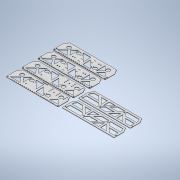
# Autodesk Inventor part: Jsun Chassi Cutout Only Outside
Saved by Autodesk Inventor 2021 (Build 250183000, 183)
## iProperties
Created: 2020-10-31
Part Number: Jsun Chassi Cutout Only Outside
Material: Generic
Document SubType Name: Modeling
Designer: deli
Density: 1 g/cm^3
Appearance: Default
Author: deli
Autodesk Inventor part; units mm, degrees
ref_plane "YZ Plane" through (0, 0, 0) normal (1, 0, 0) x (0, 1, 0)
ref_plane "XZ Plane" through (0, 0, 0) normal (0, 1, 0) x (-1, 0, 0)
ref_plane "XY Plane" through (0, 0, 0) normal (0, 0, 1) x (1, 0, 0)
sketch "Sketch1" plane through (0, 0, 0) normal (0, 1, 0) x (-1, 0, 0)
  line L0 (21, 21.4009) -> (-995, 21.4009)
  line L1 (-995, 21.4009) -> (-995, -486.5991)
  line L2 (-995, -486.5991) -> (21, -486.5991)
  line L3 (21, -486.5991) -> (21, 21.4009)
  point P0 (0, 0)
  dimension "d0" = 1016
  dimension "d1" = 508
  constraints: 8 end point, 2 parallel, 1 horizontal, 1 perpendicular
  measures "d0" distance of L2.end L1.end
  measures "d1" distance of L1.end L0.end
extrude "Extrusion1" add sketch "Sketch1" along normal blind 3.175
sketch "Sketch2" plane through (0, 3.175, 0) normal (0, 1, 0) x (1, 0, 0)
  line L0 (548.8088, 46.8923) -> (501.9154, 93.7857)
  line L1 (501.9154, 93.7857) -> (548.8088, 93.7857)
  line L2 (548.8088, 93.7857) -> (548.8088, 46.8923)
  line L3 (686.6568, 13.7857) -> (636.4088, 13.7857)
  line L4 (636.4088, 13.7857) -> (686.6568, 61.3603)
  line L5 (686.6568, 61.3603) -> (686.6568, 13.7857)
  line L6 (807.6588, 61.2857) -> (722.2634, 61.2857)
  line L7 (722.2634, 61.2857) -> (701.6568, 81.8923)
  line L8 (701.6568, 81.8923) -> (701.6568, 93.7857)
  line L9 (701.6568, 93.7857) -> (796.2302, 93.7857)
  line L10 (796.2302, 93.7857) -> (807.6588, 73.7857)
  line L11 (807.6588, 73.7857) -> (807.6588, 61.2857)
  line L12 (686.6568, 93.7857) -> (686.6568, 81.8923)
  line L13 (686.6568, 81.8923) -> (666.0502, 61.2857)
  line L14 (666.0502, 61.2857) -> (599.4154, 61.2857)
  line L15 (599.4154, 61.2857) -> (631.9154, 93.7857)
  line L16 (631.9154, 93.7857) -> (686.6568, 93.7857)
  line L17 (442.6815, 93.7857) -> (480.7022, 93.7857)
  line L18 (480.7022, 93.7857) -> (513.2022, 61.2857)
  line L19 (513.2022, 61.2857) -> (431.2588, 61.2857)
  line L20 (431.2588, 61.2857) -> (431.2588, 73.7857)
  line L21 (431.2588, 73.7857) -> (442.6815, 93.7857)
  line L22 (563.8088, 93.7857) -> (610.7022, 93.7857)
  line L23 (610.7022, 93.7857) -> (563.8088, 46.8923)
  line L24 (563.8088, 46.8923) -> (563.8088, 93.7857)
  line L25 (701.6568, 13.7857) -> (701.6568, 60.6791)
  line L26 (701.6568, 60.6791) -> (748.5502, 13.7857)
  line L27 (748.5502, 13.7857) -> (701.6568, 13.7857)
  line L28 (807.6588, 13.7857) -> (769.7634, 13.7857)
  line L29 (769.7634, 13.7857) -> (737.2634, 46.2857)
  line L30 (737.2634, 46.2857) -> (807.6588, 46.2857)
  line L31 (807.6588, 46.2857) -> (807.6588, 13.7857)
  line L32 (563.8088, 13.7857) -> (563.8088, 25.6791)
  line L33 (563.8088, 25.6791) -> (584.4154, 46.2857)
  line L34 (584.4154, 46.2857) -> (651.0502, 46.2857)
  line L35 (651.0502, 46.2857) -> (618.5502, 13.7857)
  line L36 (618.5502, 13.7857) -> (563.8088, 13.7857)
  line L37 (548.8088, 13.7857) -> (431.2588, 13.7857)
  line L38 (431.2588, 13.7857) -> (431.2588, 46.2857)
  line L39 (431.2588, 46.2857) -> (528.2022, 46.2857)
  line L40 (528.2022, 46.2857) -> (548.8088, 25.6791)
  line L41 (548.8088, 25.6791) -> (548.8088, 13.7857)
  circle A0 centre (556.3088, 28.7857) radius 3.5
  circle A1 centre (694.1568, 78.7857) radius 3.5
  circle A2 centre (423.1288, 20.1607) radius 3.5
  circle A3 centre (815.7882, 20.1789) radius 3.5
  line L42 (419.4482, -1.2143) -> (819.4793, -1.2143)
  line L43 (819.4793, -1.2143) -> (822.6588, 4.2927)
  line L44 (822.6588, 4.2927) -> (822.6588, 73.7857)
  line L45 (822.6588, 73.7857) -> (802.6588, 108.7857)
  line L46 (802.6588, 108.7857) -> (436.2486, 108.7857)
  line L47 (436.2486, 108.7857) -> (416.2588, 73.7857)
  line L48 (416.2588, 73.7857) -> (416.2588, 4.3099)
  line L49 (416.2588, 4.3099) -> (419.4482, -1.2143)
  line L50 (822.6588, 200.7857) -> (802.6588, 235.7857)
  line L51 (610.7022, 220.7857) -> (563.8088, 173.8923)
  line L52 (563.8088, 220.7857) -> (610.7022, 220.7857)
  line L53 (563.8088, 173.8923) -> (563.8088, 220.7857)
  line L54 (618.5502, 140.7857) -> (563.8088, 140.7857)
  line L55 (563.8088, 152.6791) -> (584.4154, 173.2857)
  line L56 (563.8088, 140.7857) -> (563.8088, 152.6791)
  circle A4 centre (556.3088, 155.7857) radius 3.5
  line L57 (548.8088, 152.6791) -> (548.8088, 140.7857)
  line L58 (528.2022, 173.2857) -> (548.8088, 152.6791)
  line L59 (548.8088, 220.7857) -> (548.8088, 173.8923)
  line L60 (548.8088, 173.8923) -> (501.9154, 220.7857)
  line L61 (501.9154, 220.7857) -> (548.8088, 220.7857)
  line L62 (480.7022, 220.7857) -> (513.2022, 188.2857)
  line L63 (442.6815, 220.7857) -> (480.7022, 220.7857)
  line L64 (548.8088, 140.7857) -> (431.2588, 140.7857)
  line L65 (431.2588, 173.2857) -> (528.2022, 173.2857)
  line L66 (513.2022, 188.2857) -> (431.2588, 188.2857)
  line L67 (431.2588, 188.2857) -> (431.2588, 200.7857)
  line L68 (431.2588, 140.7857) -> (431.2588, 173.2857)
  circle A5 centre (423.1288, 147.1607) radius 3.5
  line L69 (416.2588, 131.3099) -> (419.4482, 125.7857)
  line L70 (416.2588, 200.7857) -> (416.2588, 131.3099)
  line L71 (436.2486, 235.7857) -> (416.2588, 200.7857)
  line L72 (431.2588, 200.7857) -> (442.6815, 220.7857)
  line L73 (796.2302, 220.7857) -> (807.6588, 200.7857)
  line L74 (807.6588, 200.7857) -> (807.6588, 188.2857)
  circle A6 centre (815.7882, 147.1789) radius 3.5
  line L75 (822.6588, 131.2927) -> (822.6588, 200.7857)
  line L76 (819.4793, 125.7857) -> (822.6588, 131.2927)
  line L77 (807.6588, 173.2857) -> (807.6588, 140.7857)
  line L78 (737.2634, 173.2857) -> (807.6588, 173.2857)
  line L79 (807.6588, 140.7857) -> (769.7634, 140.7857)
  line L80 (807.6588, 188.2857) -> (722.2634, 188.2857)
  line L81 (701.6568, 220.7857) -> (796.2302, 220.7857)
  line L82 (769.7634, 140.7857) -> (737.2634, 173.2857)
  line L83 (722.2634, 188.2857) -> (701.6568, 208.8923)
  line L84 (701.6568, 187.6791) -> (748.5502, 140.7857)
  line L85 (748.5502, 140.7857) -> (701.6568, 140.7857)
  line L86 (701.6568, 140.7857) -> (701.6568, 187.6791)
  line L87 (701.6568, 208.8923) -> (701.6568, 220.7857)
  line L88 (599.4154, 188.2857) -> (631.9154, 220.7857)
  line L89 (584.4154, 173.2857) -> (651.0502, 173.2857)
  line L90 (802.6588, 235.7857) -> (436.2486, 235.7857)
  line L91 (419.4482, 125.7857) -> (819.4793, 125.7857)
  line L92 (666.0502, 188.2857) -> (599.4154, 188.2857)
  line L93 (651.0502, 173.2857) -> (618.5502, 140.7857)
  line L94 (631.9154, 220.7857) -> (686.6568, 220.7857)
  line L95 (686.6568, 140.7857) -> (636.4088, 140.7857)
  line L96 (636.4088, 140.7857) -> (686.6568, 188.3603)
  line L97 (686.6568, 188.3603) -> (686.6568, 140.7857)
  line L98 (686.6568, 208.8923) -> (666.0502, 188.2857)
  line L99 (686.6568, 220.7857) -> (686.6568, 208.8923)
  circle A7 centre (694.1568, 205.7857) radius 3.5
  circle A8 centre (367.8668, 73.0303) radius 2
  circle A9 centre (367.8668, 81.0303) radius 2
  circle A10 centre (367.8668, 65.0303) radius 2
  circle A11 centre (367.8668, 89.0303) radius 2
  circle A12 centre (367.8668, 57.0303) radius 2
  line L100 (185.8606, 84.0272) -> (190.0041, 79.8837)
  line L101 (190.0041, 79.8837) -> (190.0041, 23.4497)
  line L102 (190.0041, 23.4497) -> (129.4266, 84.0272)
  line L103 (129.4266, 84.0272) -> (185.8606, 84.0272)
  line L104 (205.0041, 64.8837) -> (265.5816, 4.3062)
  line L105 (265.5816, 4.3062) -> (209.1476, 4.3062)
  line L106 (209.1476, 4.3062) -> (205.0041, 8.4497)
  line L107 (205.0041, 8.4497) -> (205.0041, 64.8837)
  line L108 (93.7196, 15.6062) -> (59.7512, 53.8845)
  line L109 (59.7512, 53.8845) -> (93.7196, 84.0272)
  line L110 (93.7196, 84.0272) -> (93.7196, 15.6062)
  line L111 (312.2569, 4.3062) -> (346.6857, 38.2085)
  line L112 (346.6857, 38.2085) -> (380.0696, 4.3062)
  line L113 (380.0696, 4.3062) -> (312.2569, 4.3062)
  line L114 (3.8839, 4.3093) -> (48.5317, 43.9286)
  line L115 (48.5317, 43.9286) -> (83.6949, 4.3093)
  line L116 (83.6949, 4.3093) -> (3.8839, 4.3093)
  circle A13 centre (311.8668, 73.0303) radius 2
  circle A14 centre (255.8668, 65.0303) radius 2
  circle A15 centre (207.8668, 94.0303) radius 2
  circle A16 centre (175.8668, 94.0303) radius 2
  circle A17 centre (199.8668, 94.0303) radius 2
  circle A18 centre (255.8668, 73.0303) radius 2
  circle A19 centre (311.8668, 81.0303) radius 2
  circle A20 centre (311.8668, 65.0303) radius 2
  circle A21 centre (255.8668, 57.0303) radius 2
  circle A22 centre (255.8668, 81.0303) radius 2
  circle A23 centre (183.8668, 94.0303) radius 2
  circle A24 centre (191.8668, 94.0303) radius 2
  circle A25 centre (255.8668, 89.0303) radius 2
  circle A26 centre (311.8668, 89.0303) radius 2
  circle A27 centre (311.8668, 57.0303) radius 2
  circle A28 centre (113.7219, 19.0303) radius 3.5
  circle A29 centre (281.5699, 69.0303) radius 3.5
  circle A30 centre (-4.4581, -4.5947) radius 3.5
  circle A31 centre (388.2013, -4.5765) radius 3.5
  circle A32 centre (271.8769, -6.9697) radius 2
  circle A33 centre (143.8769, -6.9697) radius 2
  circle A34 centre (47.8769, -6.9697) radius 2
  circle A35 centre (175.8769, -6.9697) radius 2
  circle A36 centre (303.8769, -6.9697) radius 2
  circle A37 centre (239.8769, -6.9697) radius 2
  circle A38 centre (111.8769, -6.9697) radius 2
  circle A39 centre (79.8769, -6.9697) radius 2
  circle A40 centre (207.8769, -6.9697) radius 2
  circle A41 centre (335.8769, -6.9697) radius 2
  circle A42 centre (95.8769, -6.9697) radius 2
  circle A43 centre (223.8769, -6.9697) radius 2
  circle A44 centre (351.8769, -6.9697) radius 2
  circle A45 centre (255.8769, -6.9697) radius 2
  circle A46 centre (127.8769, -6.9697) radius 2
  circle A47 centre (63.8769, -6.9697) radius 2
  circle A48 centre (191.8769, -6.9697) radius 2
  circle A49 centre (319.8769, -6.9697) radius 2
  circle A50 centre (287.8769, -6.9697) radius 2
  circle A51 centre (159.8769, -6.9697) radius 2
  circle A52 centre (31.8769, -6.9697) radius 2
  circle A53 centre (345.0719, 64.0303) radius 14.275
  circle A54 centre (133.4289, 72.0303) radius 1.85
  circle A55 centre (261.8629, 32.0303) radius 1.85
  circle A56 centre (38.6719, 64.0303) radius 14.275
  circle A57 centre (253.8629, 24.0303) radius 1.85
  circle A58 centre (281.5699, 24.0303) radius 14.275
  circle A59 centre (261.8629, 16.0303) radius 1.85
  circle A60 centre (113.7219, 64.0303) radius 14.275
  circle A61 centre (141.4289, 64.0303) radius 1.85
  circle A62 centre (133.4289, 56.0303) radius 1.85
  line L117 (-11.3281, -5.4455) -> (-8.1387, -10.9697)
  line L118 (-8.1387, -10.9697) -> (391.8924, -10.9697)
  line L119 (391.8924, -10.9697) -> (395.0719, 0.8873)
  line L120 (395.0719, 0.8873) -> (395.0719, 64.0303)
  line L121 (395.0719, 64.0303) -> (375.0719, 99.0303)
  line L122 (375.0719, 99.0303) -> (8.6617, 99.0303)
  line L123 (8.6617, 99.0303) -> (-11.3281, 64.0303)
  line L124 (-11.3281, 64.0303) -> (-11.3281, -5.4455)
  line L125 (395.0719, 184.6803) -> (375.0719, 219.6803)
  circle A63 centre (367.8668, 193.6803) radius 2
  circle A64 centre (367.8668, 201.6803) radius 2
  circle A65 centre (367.8668, 209.6803) radius 2
  circle A66 centre (367.8668, 185.6803) radius 2
  circle A67 centre (367.8668, 177.6803) radius 2
  circle A68 centre (345.0719, 184.6803) radius 14.275
  circle A69 centre (311.8668, 209.6803) radius 2
  circle A70 centre (311.8668, 201.6803) radius 2
  circle A71 centre (311.8668, 193.6803) radius 2
  circle A72 centre (311.8668, 185.6803) radius 2
  circle A73 centre (311.8668, 177.6803) radius 2
  circle A74 centre (133.4289, 192.6803) radius 1.85
  circle A75 centre (133.4289, 176.6803) radius 1.85
  circle A76 centre (143.8769, 113.6803) radius 2
  circle A77 centre (159.8769, 113.6803) radius 2
  circle A78 centre (175.8769, 113.6803) radius 2
  circle A79 centre (191.8769, 113.6803) radius 2
  line L126 (129.4266, 204.6772) -> (185.8606, 204.6772)
  line L127 (190.0041, 144.0997) -> (129.4266, 204.6772)
  line L128 (190.0041, 200.5337) -> (190.0041, 144.0997)
  circle A80 centre (127.8769, 113.6803) radius 2
  circle A81 centre (113.7219, 139.6803) radius 3.5
  circle A82 centre (113.7219, 184.6803) radius 14.275
  line L129 (375.0719, 219.6803) -> (8.6617, 219.6803)
  line L130 (-8.1387, 109.6803) -> (391.8924, 109.6803)
  circle A83 centre (111.8769, 113.6803) radius 2
  circle A84 centre (141.4289, 184.6803) radius 1.85
  line L131 (185.8606, 204.6772) -> (190.0041, 200.5337)
  circle A85 centre (183.8668, 214.6803) radius 2
  circle A86 centre (191.8668, 214.6803) radius 2
  circle A87 centre (199.8668, 214.6803) radius 2
  circle A88 centre (207.8668, 214.6803) radius 2
  circle A89 centre (175.8668, 214.6803) radius 2
  line L132 (93.7196, 204.6772) -> (93.7196, 136.2562)
  line L133 (93.7196, 136.2562) -> (59.7512, 174.5345)
  line L134 (59.7512, 174.5345) -> (93.7196, 204.6772)
  line L135 (3.8839, 124.9593) -> (48.5317, 164.5786)
  line L136 (83.6949, 124.9593) -> (3.8839, 124.9593)
  line L137 (48.5317, 164.5786) -> (83.6949, 124.9593)
  circle A90 centre (95.8769, 113.6803) radius 2
  circle A91 centre (79.8769, 113.6803) radius 2
  circle A92 centre (63.8769, 113.6803) radius 2
  circle A93 centre (47.8769, 113.6803) radius 2
  circle A94 centre (31.8769, 113.6803) radius 2
  circle A95 centre (-4.4581, 116.0553) radius 3.5
  line L138 (-11.3281, 115.2045) -> (-8.1387, 109.6803)
  line L139 (-11.3281, 184.6803) -> (-11.3281, 115.2045)
  line L140 (8.6617, 219.6803) -> (-11.3281, 184.6803)
  circle A96 centre (38.6719, 184.6803) radius 14.275
  line L141 (395.0719, 121.5373) -> (395.0719, 184.6803)
  line L142 (346.6857, 158.8585) -> (380.0696, 124.9562)
  line L143 (312.2569, 124.9562) -> (346.6857, 158.8585)
  line L144 (380.0696, 124.9562) -> (312.2569, 124.9562)
  circle A97 centre (319.8769, 113.6803) radius 2
  circle A98 centre (335.8769, 113.6803) radius 2
  circle A99 centre (351.8769, 113.6803) radius 2
  circle A100 centre (388.2013, 116.0735) radius 3.5
  line L145 (391.8924, 109.6803) -> (395.0719, 121.5373)
  circle A101 centre (303.8769, 113.6803) radius 2
  circle A102 centre (287.8769, 113.6803) radius 2
  circle A103 centre (271.8769, 113.6803) radius 2
  circle A104 centre (281.5699, 144.6803) radius 14.275
  circle A105 centre (281.5699, 189.6803) radius 3.5
  circle A106 centre (255.8668, 185.6803) radius 2
  circle A107 centre (255.8668, 177.6803) radius 2
  circle A108 centre (255.8668, 193.6803) radius 2
  circle A109 centre (255.8668, 201.6803) radius 2
  circle A110 centre (255.8668, 209.6803) radius 2
  circle A111 centre (261.8629, 152.6803) radius 1.85
  circle A112 centre (261.8629, 136.6803) radius 1.85
  circle A113 centre (253.8629, 144.6803) radius 1.85
  circle A114 centre (255.8769, 113.6803) radius 2
  line L146 (209.1476, 124.9562) -> (205.0041, 129.0997)
  circle A115 centre (207.8769, 113.6803) radius 2
  line L147 (265.5816, 124.9562) -> (209.1476, 124.9562)
  line L148 (205.0041, 185.5337) -> (265.5816, 124.9562)
  circle A116 centre (223.8769, 113.6803) radius 2
  circle A117 centre (239.8769, 113.6803) radius 2
  line L149 (205.0041, 129.0997) -> (205.0041, 185.5337)
  line L150 (209.0752, 250.5034) -> (204.9317, 254.6469)
  line L151 (204.9317, 254.6469) -> (204.9317, 311.0809)
  line L152 (204.9317, 311.0809) -> (265.5092, 250.5034)
  line L153 (265.5092, 250.5034) -> (209.0752, 250.5034)
  line L154 (59.6793, 300.0817) -> (93.6472, 330.2244)
  line L155 (93.6472, 330.2244) -> (93.6472, 261.8031)
  line L156 (93.6472, 261.8031) -> (59.6793, 300.0817)
  line L157 (301.4952, 330.2244) -> (336.0887, 295.0937)
  line L158 (336.0887, 295.0937) -> (301.4952, 261.0292)
  line L159 (301.4952, 261.0292) -> (301.4952, 330.2244)
  line L160 (129.3542, 330.2244) -> (185.7882, 330.2244)
  line L161 (185.7882, 330.2244) -> (189.9317, 326.0809)
  line L162 (189.9317, 326.0809) -> (189.9317, 269.6469)
  line L163 (189.9317, 269.6469) -> (129.3542, 330.2244)
  line L164 (83.6201, 250.5034) -> (3.8092, 250.5034)
  line L165 (3.8092, 250.5034) -> (48.4598, 290.1257)
  line L166 (48.4598, 290.1257) -> (83.6201, 250.5034)
  line L167 (346.6133, 284.4057) -> (379.9972, 250.5034)
  line L168 (379.9972, 250.5034) -> (312.1845, 250.5034)
  line L169 (312.1845, 250.5034) -> (346.6133, 284.4057)
  circle A118 centre (281.4952, 315.2244) radius 3.5
  circle A119 centre (-4.5328, 241.5994) radius 3.5
  circle A120 centre (128.6472, 265.2244) radius 3.5
  circle A121 centre (388.1266, 256.6176) radius 3.5
  circle A122 centre (266.4952, 315.2244) radius 3.5
  circle A123 centre (-4.5328, 256.5994) radius 3.5
  circle A124 centre (113.6472, 265.2244) radius 3.5
  circle A125 centre (388.1266, 241.6176) radius 3.5
  circle A126 centre (271.8022, 239.2244) radius 2
  circle A127 centre (143.8022, 239.2244) radius 2
  circle A128 centre (47.8022, 239.2244) radius 2
  circle A129 centre (175.8022, 239.2244) radius 2
  circle A130 centre (303.8022, 239.2244) radius 2
  circle A131 centre (239.8022, 239.2244) radius 2
  circle A132 centre (111.8022, 239.2244) radius 2
  circle A133 centre (79.8022, 239.2244) radius 2
  circle A134 centre (207.8022, 239.2244) radius 2
  circle A135 centre (335.8022, 239.2244) radius 2
  circle A136 centre (287.8022, 239.2244) radius 2
  circle A137 centre (159.8022, 239.2244) radius 2
  circle A138 centre (31.8022, 239.2244) radius 2
  circle A139 centre (127.8022, 239.2244) radius 2
  circle A140 centre (255.8022, 239.2244) radius 2
  circle A141 centre (319.8022, 239.2244) radius 2
  circle A142 centre (191.8022, 239.2244) radius 2
  circle A143 centre (63.8022, 239.2244) radius 2
  circle A144 centre (95.8022, 239.2244) radius 2
  circle A145 centre (223.8022, 239.2244) radius 2
  circle A146 centre (351.8022, 239.2244) radius 2
  circle A147 centre (233.0022, 298.2244) radius 1.85
  circle A148 centre (171.1402, 258.2244) radius 1.85
  circle A149 centre (171.1402, 282.2244) radius 1.85
  circle A150 centre (224.0022, 322.2244) radius 1.85
  circle A151 centre (224.0022, 298.2244) radius 1.85
  circle A152 centre (162.1402, 258.2244) radius 1.85
  circle A153 centre (162.1402, 282.2244) radius 1.85
  circle A154 centre (233.0022, 322.2244) radius 1.85
  circle A155 centre (344.9972, 310.2244) radius 14.275
  circle A156 centre (133.3542, 318.2244) radius 1.85
  circle A157 centre (261.7882, 278.2244) radius 1.85
  circle A158 centre (38.5972, 310.2244) radius 14.275
  circle A159 centre (253.7882, 270.2244) radius 1.85
  circle A160 centre (281.4952, 270.2244) radius 14.275
  circle A161 centre (261.7882, 262.2244) radius 1.85
  circle A162 centre (113.6472, 310.2244) radius 14.275
  circle A163 centre (141.3542, 310.2244) radius 1.85
  circle A164 centre (133.3542, 302.2244) radius 1.85
  line L170 (-11.4028, 240.7486) -> (-8.2134, 235.2244)
  line L171 (-8.2134, 235.2244) -> (391.8178, 235.2244)
  line L172 (391.8178, 235.2244) -> (394.9972, 240.7314)
  line L173 (394.9972, 240.7314) -> (394.9972, 310.2244)
  line L174 (394.9972, 310.2244) -> (374.9972, 345.2244)
  line L175 (374.9972, 345.2244) -> (8.587, 345.2244)
  line L176 (8.587, 345.2244) -> (-11.4028, 310.2244)
  line L177 (-11.4028, 310.2244) -> (-11.4028, 240.7486)
  circle A165 centre (127.8022, 359.8744) radius 2
  line L178 (209.0752, 371.1534) -> (204.9317, 375.2969)
  line L179 (265.5092, 371.1534) -> (209.0752, 371.1534)
  line L180 (204.9317, 375.2969) -> (204.9317, 431.7309)
  line L181 (-8.2134, 355.8744) -> (391.8178, 355.8744)
  line L182 (374.9972, 465.8744) -> (8.587, 465.8744)
  line L183 (204.9317, 431.7309) -> (265.5092, 371.1534)
  circle A166 centre (253.7882, 390.8744) radius 1.85
  circle A167 centre (191.8022, 359.8744) radius 2
  circle A168 centre (207.8022, 359.8744) radius 2
  circle A169 centre (223.8022, 359.8744) radius 2
  circle A170 centre (224.0022, 418.8744) radius 1.85
  circle A171 centre (224.0022, 442.8744) radius 1.85
  circle A172 centre (233.0022, 442.8744) radius 1.85
  circle A173 centre (233.0022, 418.8744) radius 1.85
  circle A174 centre (239.8022, 359.8744) radius 2
  circle A175 centre (287.8022, 359.8744) radius 2
  circle A176 centre (303.8022, 359.8744) radius 2
  circle A177 centre (162.1402, 378.8744) radius 1.85
  circle A178 centre (171.1402, 378.8744) radius 1.85
  circle A179 centre (143.8022, 359.8744) radius 2
  circle A180 centre (175.8022, 359.8744) radius 2
  circle A181 centre (159.8022, 359.8744) radius 2
  circle A182 centre (162.1402, 402.8744) radius 1.85
  circle A183 centre (133.3542, 422.8744) radius 1.85
  circle A184 centre (141.3542, 430.8744) radius 1.85
  circle A185 centre (133.3542, 438.8744) radius 1.85
  line L184 (129.3542, 450.8744) -> (185.7882, 450.8744)
  line L185 (189.9317, 390.2969) -> (129.3542, 450.8744)
  line L186 (189.9317, 446.7309) -> (189.9317, 390.2969)
  line L187 (185.7882, 450.8744) -> (189.9317, 446.7309)
  circle A186 centre (171.1402, 402.8744) radius 1.85
  circle A187 centre (128.6472, 385.8744) radius 3.5
  circle A188 centre (113.6472, 430.8744) radius 14.275
  circle A189 centre (113.6472, 385.8744) radius 3.5
  circle A190 centre (111.8022, 359.8744) radius 2
  circle A191 centre (95.8022, 359.8744) radius 2
  circle A192 centre (38.5972, 430.8744) radius 14.275
  circle A193 centre (31.8022, 359.8744) radius 2
  line L188 (-11.4028, 361.3986) -> (-8.2134, 355.8744)
  line L189 (-11.4028, 430.8744) -> (-11.4028, 361.3986)
  circle A194 centre (-4.5328, 377.2494) radius 3.5
  line L190 (8.587, 465.8744) -> (-11.4028, 430.8744)
  line L191 (93.6472, 450.8744) -> (93.6472, 382.4531)
  line L192 (59.6793, 420.7317) -> (93.6472, 450.8744)
  line L193 (93.6472, 382.4531) -> (59.6793, 420.7317)
  line L194 (83.6201, 371.1534) -> (3.8092, 371.1534)
  line L195 (3.8092, 371.1534) -> (48.4598, 410.7757)
  circle A195 centre (-4.5328, 362.2494) radius 3.5
  line L196 (48.4598, 410.7757) -> (83.6201, 371.1534)
  circle A196 centre (47.8022, 359.8744) radius 2
  circle A197 centre (63.8022, 359.8744) radius 2
  circle A198 centre (79.8022, 359.8744) radius 2
  line L197 (336.0887, 415.7437) -> (301.4952, 381.6792)
  circle A199 centre (271.8022, 359.8744) radius 2
  line L198 (379.9972, 371.1534) -> (312.1845, 371.1534)
  circle A200 centre (255.8022, 359.8744) radius 2
  circle A201 centre (388.1266, 362.2676) radius 3.5
  circle A202 centre (261.7882, 382.8744) radius 1.85
  circle A203 centre (261.7882, 398.8744) radius 1.85
  circle A204 centre (266.4952, 435.8744) radius 3.5
  circle A205 centre (281.4952, 435.8744) radius 3.5
  circle A206 centre (281.4952, 390.8744) radius 14.275
  line L199 (312.1845, 371.1534) -> (346.6133, 405.0557)
  line L200 (346.6133, 405.0557) -> (379.9972, 371.1534)
  line L201 (301.4952, 381.6792) -> (301.4952, 450.8744)
  line L202 (301.4952, 450.8744) -> (336.0887, 415.7437)
  circle A207 centre (335.8022, 359.8744) radius 2
  circle A208 centre (319.8022, 359.8744) radius 2
  circle A209 centre (351.8022, 359.8744) radius 2
  circle A210 centre (344.9972, 430.8744) radius 14.275
  line L203 (391.8178, 355.8744) -> (394.9972, 361.3814)
  line L204 (394.9972, 430.8744) -> (374.9972, 465.8744)
  line L205 (394.9972, 361.3814) -> (394.9972, 430.8744)
  circle A211 centre (388.1266, 377.2676) radius 3.5
  line L206 (995, -21.4009) -> (995, 486.5991) projected
  line L207 (995, 486.5991) -> (-21, 486.5991) projected
  line L208 (-21, 486.5991) -> (-21, -21.4009) projected
  line L209 (-21, -21.4009) -> (995, -21.4009) projected
  point P0 (0, 0)
  point P1 (822.6588, 73.7857)
  point P2 (822.6588, 200.7857)
  point P3 (395.0719, 64.0303)
  point P4 (395.0719, 184.6803)
  point P5 (394.9972, 310.2244)
  point P6 (394.9972, 430.8744)
  dimension "d6" = 127
  dimension "d13" = 120.65
  dimension "d20" = 120.65
  constraints: 412 end point, 212 centre point, 3 collinear, 3 vertical, 418 other
  measures "d6" distance of L10.end L73.end
  measures "d13" distance of L121.start L125.start
  measures "d20" distance of A139.centre A165.centre
extrude "Extrusion3" cut sketch "Sketch2" against normal blind 25.4
body "Solid1"
